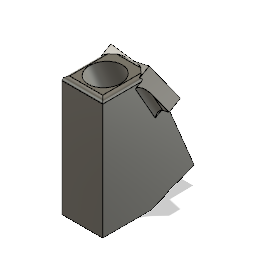
57part (Autodesk Fusion 360 design; units mm, degrees)
Autodesk Fusion 360 part; units mm, degrees
note: some values were not read from the file. Set by a fixed rule: which face or edge a step refers to.
sketch "Sketch1" plane through (0, 0, 0) normal (1, 0, 0) x (0, 0, -1)
  line L0 (210, 530.000008) -> (260.310359, 530.000008)
  line L1 (260.310359, 530.000008) -> (303.817128, 425.188246)
  line L2 (303.817128, 425.188246) -> (260.000004, 407.000006)
  line L3 (260.000004, 407.000006) -> (210, 407.000006)
  line L4 (210, 407.000006) -> (210, 530.000008)
  line L5 (178.612871, 686.943083) -> (561.990543, -236.648581)
  constraint horizontal L0
  constraint perpendicular L1 L2
  constraint parallel L0 L3
  constraint perpendicular L0 L4
  constraint parallel L1 L5
extrude "Extrude1" add sketch "Sketch1" along normal mid plane 42 contours L0 L2 L3 L4 L5 | L0 L1 L2 L5 picked at (237.919686, 448.000007) picked at (264.589307, 493.109234)
ref_plane "WorkPlane1" through (0, 416.094126, -281.908566) normal (0, 0.923592, 0.383378) x (0, -0.383378, 0.923592)
sketch "Sketch2" plane through (0, 416.094126, -281.908566) normal (0, 0.923592, 0.383378) x (0, -0.383378, 0.923592)
  circle A0 centre (1, 0) radius 16
  dimension "d8" = 32
  measures "d8" diameter of A0
extrude "Extrude3" cut sketch "Sketch2" along normal mid plane 300 contours A0 picked at (5.030821, 7.451498)
chamfer "Chamfer1" distance 6 angle 45 1 edges at (-5.785847, 421.429684, -294.76241)
fillet "Fillet3" radius 4 4 edges at (21, 530.000008, -235.15518) (0, 530.000008, -260.310359) (-21, 530.000008, -235.15518) (0, 530.000008, -210)
sketch "Sketch3" plane through (145.776668, 58.614343, 32.64009) normal (-0.908414, -0.365258, -0.203398) x (-0.218495, 0, 0.975838)
  line L0 (-547.70817, 44.463109) -> (-536.246231, 37.330511)
  line L1 (-536.246231, 37.330511) -> (-245.658923, 504.298408)
  line L2 (-245.658923, 504.298408) -> (-257.120862, 511.431005)
  line L3 (-257.120862, 511.431005) -> (-547.70817, 44.463109)
  line L4 (-547.70817, 44.463109) -> (-536.246231, 37.330511)
  line L5 (-536.246231, 37.330511) -> (-245.658923, 504.298408)
  line L6 (-245.658923, 504.298408) -> (-257.120862, 511.431005)
  line L7 (-257.120862, 511.431005) -> (-547.70817, 44.463109)
  line L8 (-257.120862, 511.431005) -> (-245.658923, 504.298408)
  line L9 (-245.658923, 504.298408) -> (-265.229974, 472.848125)
  line L10 (-265.229974, 472.848125) -> (-276.691914, 479.980723)
  line L11 (-276.691914, 479.980723) -> (-257.120862, 511.431005)
  constraint perpendicular L8 L9
  constraint parallel L8 L10
  constraint parallel L9 L11
extrude "Extrude4" add sketch "Sketch3" along normal blind 20 contours L1 L2 L3 L5 L6 L7 L8 L9 L10 L11 picked at (-266.347583, 488.086618)
mirror "Mirror1" about plane through (0, 0, 0) normal (1, 0, 0) of "Extrude4"
fillet "Fillet4" radius 6 8 edges at (-9.250715, 510.943019, -268.220807) (-18.999775, 496.146148, -274.362904) (-21, 495.044499, -270.551229) (18.999775, 496.146148, -274.362904) (-21, 509.35203, -257.906843) (21, 495.044499, -270.551229) (21, 509.35203, -257.906843) (9.250715, 510.943019, -268.220807)
delete_face "DeleteFace1" 1 faces at (-3.884147, 522.494531, -252.259524)
delete_face "DeleteFace2" 1 faces at (2.348814, 522.027039, -252.867751)
